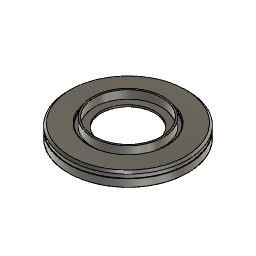
TouchCap (Autodesk Fusion 360 design; units mm, degrees)
Autodesk Fusion 360 part; units mm, degrees
sketch "Sketch2" plane through (0, 0, 0) normal (0, 1, 0) x (1, 0, 0) in component "LensCap_Sony20mm"
  line L0 (18.85, -1.2) -> (22.35, -1.2)
  line L1 (22.35, -1.2) -> (22.35, 0)
  line L2 (22.35, 0) -> (26, 0)
  line L3 (26, 0) -> (26, -2.7)
  line L4 (26, -2.7) -> (18.85, -2.7)
  line L5 (18.85, -2.7) -> (18.85, -1.2)
  line L6 (17.35, -5.2) -> (17.35, -1.2)
  line L7 (17.35, -1.2) -> (20.85, -1.2)
  line L8 (20.85, -1.2) -> (20.85, -0.2)
  line L9 (20.85, -0.2) -> (13.25, -0.2)
  line L10 (13.25, -0.2) -> (13.25, -1.2)
  line L11 (13.25, -1.2) -> (16.55, -1.2)
  line L12 (16.55, -1.2) -> (16.55, -5.2)
  line L13 (16.55, -5.2) -> (17.35, -5.2)
  line L14 (0, 0) -> (0, -2.7)
  line L15 (22.35, 0) -> (0, 0)
  line L16 (0, -2.7) -> (18.85, -2.7)
  line L17 (18.85, 0) -> (18.85, 2)
  line L18 (18.85, 2) -> (22.45, 2)
  line L19 (22.45, 2) -> (22.45, 5)
  line L20 (22.45, 5) -> (23.65, 5)
  line L21 (23.65, 5) -> (23.65, 2)
  line L22 (23.65, 2) -> (26, 2)
  line L23 (26, 2) -> (26, 0)
  dimension "d17" = 2.7
  dimension "d18" = 1.2
  dimension "d19" = 0.8
  dimension "d20" = 1
  dimension "d21" = 16.55
  dimension "d22" = 1.5
  dimension "d24" = 3.5
  dimension "d25" = 3.3
  dimension "d26" = 4
  dimension "d33" = 1.5
  dimension "d34" = 2
  dimension "d35" = 3
  dimension "d36" = 23.65
  dimension "d37" = 1.2
  dimension "d40" = 26
  constraint horizontal L0
  constraint perpendicular L0 L1
  constraint perpendicular L1 L2
  constraint perpendicular L2 L3
  constraint perpendicular L1 L4
  constraint perpendicular L4 L5
  constraint perpendicular L0 L6
  constraint perpendicular L6 L7
  constraint perpendicular L0 L8
  constraint perpendicular L8 L9
  constraint perpendicular L9 L10
  constraint perpendicular L10 L11
  constraint perpendicular L11 L12
  constraint perpendicular L6 L13
  constraint coincident L14.start L2
  constraint coincident L6.end L11
  constraint coincident L0 L7.end
  constraint coincident L14.start L15.end
  constraint horizontal L16
  constraint vertical L14
  constraint coincident L15 L17.start
  constraint perpendicular L15 L17
  constraint perpendicular L17 L18
  constraint perpendicular L18 L19
  constraint perpendicular L19 L20
  constraint perpendicular L20 L21
  constraint perpendicular L21 L22
  constraint perpendicular L22 L23
  constraint coincident L18 L21.end
  constraint coincident L0.start L17
  measures "d17" distance of L3.end L2.end
  measures "d18" distance of L0.end L1.end
  measures "d19" distance of L6.start L12.end
  measures "d20" distance of L7.end L8.end
  measures "d21" horizontal distance of L14.start L12.end
  measures "d22" horizontal distance of L4.end L6.start
  measures "d24" horizontal distance of L6.end L8.end
  measures "d25" horizontal distance of L9.end L11.end
  measures "d26" distance of L11.end L12.end
  measures "d33" distance of L1 L8
  measures "d34" distance of L22.end L2.end
  measures "d35" distance of L20.end L21.end
  measures "d36" distance of L14.start L21
  measures "d37" distance of L19.end L20.end
  measures "d40" distance of L14.start L2.end
revolve "Revolve3" add sketch "Sketch2" angle 360 about axis through (0, 0, 1.75) along (0, 0, 1) contours L0 L1 L2 L3 L4 L5 L7 makes body 1 in component "LensCap_Sony20mm"
revolve "Revolve4" add sketch "Sketch2" angle 360 about axis through (0, 0, 1.75) along (0, 0, 1) separate body contours L2 L15 L17 L18 L19 L20 L21 L22 L23 makes body 2 in component "LensCap_Sony20mm"
revolve "Revolve5" add sketch "Sketch2" angle 360 about axis through (0, 0, 1.75) along (0, 0, 1) separate body contours L0 L6 L7 L8 L9 L10 L11 L12 L16 | L6 L12 L13 L16 makes body 3 in component "LensCap_Sony20mm"
chamfer "Chamfer5" distance 1 angle 45 1 edges at (-24.2405, -9.402, 2.7) on bodies 1 in component "LensCap_Sony20mm"
sketch "Sketch3" plane through (0, 0, 0) normal (0, 0, 1) x (1, 0, 0) in component "LensCap_Sony20mm"
  circle A0 centre (0, 0) radius 26 construction
  circle A1 centre (0, 0) radius 22.35 construction
  line L0 (22.35, 0) -> (26, 0) construction
  circle A2 centre (0, 0) radius 24.175 construction
  line L1 (0, 0) -> (0, 26) construction
  circle A3 centre (0, 24.175) radius 0.8
  circle A4 centre (-20.9362, -12.0875) radius 0.8
  circle A5 centre (20.9362, -12.0875) radius 0.8
  circle A6 centre (0, 24.175) radius 0.95
  circle A7 centre (-20.9362, -12.0875) radius 0.95
  circle A8 centre (20.9362, -12.0875) radius 0.95
  point P0 (26, 0)
  point P1 (22.35, 0)
  point P2 (24.175, 0)
  dimension "d46" = 360
  dimension "d47" = 1.6
  dimension "d48" = 0.15
  constraint coincident A0.centre A1.centre
  constraint concentric A0 A1
  constraint coincident A1 P1
  constraint coincident A0 P0
  constraint coincident P1 L0.start
  constraint coincident P0 L0.end
  constraint coincident A0 L1.end
  constraint vertical L1
  constraint midpoint L0 P2
  constraint coincident A2 P2
  constraint coincident A2 A3.centre
  constraint coincident L1 A3.centre
  measures "d47" diameter of A3
extrude "Extrude5" add sketch "Sketch3" against normal blind 1.8 contours A3 | A4 | A5 bodies 1 in component "LensCap_Sony20mm"
extrude "Extrude6" cut sketch "Sketch3" against normal up to surface (2 mm away) contours A3 | A4 | A5 | A6 | A7 | A8 bodies 2 in component "LensCap_Sony20mm"
chamfer "Chamfer9" distance 0.3 angle 45 3 edges at (0, 23.65, -2) (-20.4815, -11.825, -2) (20.4815, -11.825, -2) on bodies 2 in component "LensCap_Sony20mm"
chamfer "Chamfer10" distance 0.3 angle 45 1 edges at (-17.5744, -6.8165, 2.7) on bodies 1 in component "LensCap_Sony20mm"
chamfer "Chamfer7" distance 0.25 angle 45 1 faces at (18.239, -1.0358, 0.2) on bodies 3 in component "LensCap_Sony20mm"
chamfer "Chamfer8" distance 0.25 angle 45 1 faces at (-3.5989, 22.4717, 0) on bodies 2 in component "LensCap_Sony20mm"
sketch "Sketch1" plane through (0, 0, 0) normal (0, 1, 0) x (1, 0, 0) in component "Blob"
  line L0 (0, 0) -> (0, -24.5001)
  line L1 (-13.5, 0) -> (-13.5, -3)
  ellipse E0 centre (17.5, -12.055) end of major axis (17.5, -18.055) minor radius 2.5
  line L2 (17.5, -6.055) -> (17.5, -18.055)
  line L3 (15, -12.055) -> (20, -12.055)
  circle A0 centre (0, 5.4999) radius 30
  line L4 (-13.5, -3) -> (-10, -3)
  line L5 (-10, -3) -> (-10, -5)
  line L6 (0, 5.4999) -> (0, 0) construction
  line L7 (-10, -5) -> (0, -5)
  line L8 (-16.5, 0) -> (-13.5, 0)
  line L9 (-16.5, 0) -> (-16.5, -19.555)
  ellipse E1 centre (-17.5, -12.055) end of major axis (-17.5, -6.055) minor radius 2.5
  line L10 (-17.5, -18.055) -> (-17.5, -6.055)
  line L11 (-15, -12.055) -> (-20, -12.055)
  circle A1 centre (0, -8.5) radius 7.5
  dimension "d683" = 3
  dimension "d684" = 3.5
  dimension "d685" = 15
  dimension "d686" = 16.5
  dimension "d687" = 3
  dimension "d688" = 2
  dimension "d689" = 8.5
  dimension "d690" = 19.555
  dimension "d691" = 60
  dimension "d697" = 1
  dimension "d698" = 7.5
  dimension "d699" = 12
  dimension "d700" = 5
  constraint horizontal L8
  constraint perpendicular L1 L8
  constraint perpendicular L1 L4
  constraint perpendicular L4 L5
  constraint perpendicular L5 L7
  constraint coincident L9.end A0
  constraint perpendicular L8 L9
  constraint coincident L0.start L6.end
  constraint coincident L0.end A0
  constraint perpendicular L0 L8
  constraint coincident L7.end L0
  constraint coincident A0.centre L6.start
  constraint coincident L0.start L8
  constraint vertical L6
  constraint coincident A1.centre L0
  constraint coincident L10.start E1
  constraint coincident L10.end E1
  constraint coincident L11.start E1
  constraint coincident L11.end E1
  constraint parallel L9 L10
  constraint coincident L2.start E0
  constraint coincident L2.end E0
  constraint coincident L3.start E0
  constraint coincident L3.end E0
  constraint vertical L2
  constraint symmetric L0 L2 L10
  constraint symmetric L0 L3 L11
  constraint symmetric L10.start L2.end L0
  constraint symmetric L11.start L3.start L0
  measures "d683" distance of L8.start L1.start
  measures "d684" distance of L1.end L4.end
  measures "d685" diameter of A1
  measures "d686" distance of L8.start L0.start
  measures "d687" distance of L1.start L1.end
  measures "d688" distance of L4.end L5.end
  measures "d689" distance of A1.centre L0.start
  measures "d690" distance of L8.start L9.end
  measures "d691" diameter of A0
  measures "d697" horizontal distance of L9.end L10.start
  measures "d698" distance of L9.end E1.centre
  measures "d699" distance of E1
revolve "Revolve1" add sketch "Sketch1" angle 360 about axis through (0, 0, 0) along (0, 0, 1) separate body contours L0 L7 A1 | L0 L7 A1 | L0 L1 A0 L4 L5 L7 L8 L9 E1 A1 | L9 E1 L11 | L9 E1 L11 picked at (-11.3366, -16.9039) makes body 4 in component "Blob"
extrude "Extrude1" cut sketch "Sketch1" along normal through all and the other way through all contours L9 E1 L10 L11 | L9 E1 L11 | L9 E1 L10 L11 | L9 E1 L11 | E1 L10 L11 | E1 L10 L11 | E0 L2 L3 | E0 L2 L3 | E0 L2 L3 | E0 L2 L3 bodies 4 in component "Blob"
sketch "Sketch2 (2)" plane through (0, 0, 0) normal (0, 1, 0) x (1, 0, 0) in component "LensCap_Sony20mm_2"
  line L0 (18.6, -1.2) -> (24.4, -1.2)
  line L1 (24.4, -1.2) -> (24.4, 0)
  line L2 (24.4, 0) -> (29, 0)
  line L3 (29, 0) -> (29, -2.7)
  line L4 (29, -2.7) -> (18.6, -2.7)
  line L5 (18.6, -2.7) -> (18.6, -1.2)
  line L6 (17.1, -5.2) -> (17.1, -1.2)
  line L7 (17.1, -1.2) -> (20.4, -1.2)
  line L8 (20.4, -1.2) -> (20.4, -0.2)
  line L9 (20.4, -0.2) -> (13, -0.2)
  line L10 (13, -0.2) -> (13, -1.2)
  line L11 (13, -1.2) -> (16.3, -1.2)
  line L12 (16.3, -1.2) -> (16.3, -5.2)
  line L13 (16.3, -5.2) -> (17.1, -5.2)
  line L14 (0, 0) -> (0, -2.7)
  line L15 (24.4, 0) -> (0, 0)
  line L16 (0, -2.7) -> (18.6, -2.7)
  line L17 (18.6, 0) -> (18.6, 1)
  line L18 (18.6, 1) -> (26.65, 1)
  line L19 (26.65, 1) -> (26.65, 4)
  line L20 (26.65, 4) -> (28.25, 4)
  line L21 (28.25, 4) -> (28.25, 1)
  line L22 (28.25, 1) -> (29, 1)
  line L23 (29, 1) -> (29, 0)
  line L24 (28.25, 4) -> (29, 4)
  line L25 (29, 4) -> (29, 1)
  dimension "d17_1" = 2.7
  dimension "d18_1" = 1.2
  dimension "d19_1" = 0.8
  dimension "d20_1" = 1
  dimension "d21_1" = 16.3
  dimension "d22_1" = 1.5
  dimension "d24_1" = 3.3
  dimension "d25_1" = 3.3
  dimension "d26_1" = 4
  dimension "d33_1" = 4
  dimension "d34_1" = 1
  dimension "d35_1" = 3
  dimension "d37_1" = 1.6
  dimension "d40_1" = 29
  dimension "d77" = 26.65
  dimension "d78" = 28.25
  constraint horizontal L0
  constraint perpendicular L0 L1
  constraint perpendicular L1 L2
  constraint perpendicular L2 L3
  constraint perpendicular L1 L4
  constraint perpendicular L4 L5
  constraint perpendicular L0 L6
  constraint perpendicular L6 L7
  constraint perpendicular L0 L8
  constraint perpendicular L8 L9
  constraint perpendicular L9 L10
  constraint perpendicular L10 L11
  constraint perpendicular L11 L12
  constraint perpendicular L6 L13
  constraint coincident L14.start L2
  constraint coincident L6.end L11
  constraint coincident L0 L7.end
  constraint coincident L14.start L15.end
  constraint horizontal L16
  constraint vertical L14
  constraint coincident L15 L17.start
  constraint perpendicular L15 L17
  constraint perpendicular L17 L18
  constraint perpendicular L18 L19
  constraint perpendicular L19 L20
  constraint perpendicular L20 L21
  constraint perpendicular L21 L22
  constraint perpendicular L22 L23
  constraint coincident L18 L21.end
  constraint coincident L0.start L17
  constraint perpendicular L21 L24
  constraint perpendicular L24 L25
  measures "d17_1" distance of L3.end L2.end
  measures "d18_1" distance of L0.end L1.end
  measures "d19_1" distance of L6.start L12.end
  measures "d20_1" distance of L7.end L8.end
  measures "d21_1" horizontal distance of L14.start L12.end
  measures "d22_1" horizontal distance of L4.end L6.start
  measures "d24_1" horizontal distance of L6.end L8.end
  measures "d25_1" horizontal distance of L9.end L11.end
  measures "d26_1" distance of L11.end L12.end
  measures "d33_1" distance of L1 L8
  measures "d34_1" distance of L22.end L2.end
  measures "d35_1" distance of L20.end L21.end
  measures "d37_1" distance of L19.end L20.end
  measures "d40_1" distance of L14.start L2.end
  measures "d77" horizontal distance of L14.start L19.end
  measures "d78" horizontal distance of L14.start L20.end
revolve "Revolve3'" add sketch "Sketch2 (2)" angle 360 about axis through (0, 0, 1.75) along (0, 0, 1) separate body contours L0 L1 L2 L3 L4 L5 L7 makes body 5 in component "LensCap_Sony20mm_2"
revolve "Revolve4'" add sketch "Sketch2 (2)" angle 360 about axis through (0, 0, 1.75) along (0, 0, 1) separate body contours L2 L15 L17 L18 L19 L20 L21 L22 L23 | L21 L22 L24 L25 makes body 6 in component "LensCap_Sony20mm_2"
revolve "Revolve5'" add sketch "Sketch2 (2)" angle 360 about axis through (0, 0, 1.75) along (0, 0, 1) separate body contours L0 L6 L7 L8 L9 L10 L11 L12 L16 | L6 L12 L13 L16 makes body 7 in component "LensCap_Sony20mm_2"
chamfer "Chamfer5'" distance 1 angle 45 1 edges at (-27.0375, -10.4868, 2.7) on bodies 5 in component "LensCap_Sony20mm_2"
sketch "Sketch3 (2)" plane through (0, 0, 0) normal (0, 0, 1) x (1, 0, 0) in component "LensCap_Sony20mm_2"
  circle A0 centre (0, 0) radius 29 construction
  circle A1 centre (0, 0) radius 24.4 construction
  line L0 (24.4, 0) -> (29, 0) construction
  circle A2 centre (0, 0) radius 26.7 construction
  line L1 (0, 0) -> (0, 29) construction
  circle A3 centre (0, 0) radius 20.4
  circle A4 centre (0, 0) radius 24.8 construction
  line L2 (0, 0) -> (24.8, 0) construction
  line L3 (0, 0) -> (22.4764, -10.4809) construction
  circle A5 centre (14.2796, -6.6587) radius 9.0442 construction
  circle A6 centre (14.2796, -6.6587) radius 7.8442 construction
  circle A7 centre (21.9326, -10.2274) radius 0.6
  arc A8 (22.4764, -10.4809) -> (20.4, 0) centre (14.2796, -6.6587) ccw
  arc A9 (21.3889, -9.9738) -> (20.3317, -1.6683) centre (14.2796, -6.6587) ccw
  arc A10 (23.5102, 2.0569) -> (18.4419, 8.721) centre (15.6959, 1.3732) ccw
  arc A11 (24.7056, 2.1615) -> (17.6669, 10.2) centre (15.6959, 1.3732) ccw
  circle A12 centre (24.1079, 2.1092) radius 0.6
  arc A13 (19.332, 13.5364) -> (11.6106, 16.7736) centre (12.9064, 9.0372) ccw
  arc A14 (20.315, 14.2247) -> (10.2, 17.6669) centre (12.9064, 9.0372) ccw
  circle A15 centre (19.8235, 13.8805) radius 0.6
  arc A16 (9.9738, 21.3889) -> (1.6683, 20.3317) centre (6.6587, 14.2796) ccw
  arc A17 (10.4809, 22.4764) -> (0, 20.4) centre (6.6587, 14.2796) ccw
  circle A18 centre (10.2274, 21.9326) radius 0.6
  arc A19 (-2.0569, 23.5102) -> (-8.721, 18.4419) centre (-1.3732, 15.6959) ccw
  arc A20 (-2.1615, 24.7056) -> (-10.2, 17.6669) centre (-1.3732, 15.6959) ccw
  circle A21 centre (-2.1092, 24.1079) radius 0.6
  arc A22 (-13.5364, 19.332) -> (-16.7736, 11.6106) centre (-9.0372, 12.9064) ccw
  arc A23 (-14.2247, 20.315) -> (-17.6669, 10.2) centre (-9.0372, 12.9064) ccw
  circle A24 centre (-13.8805, 19.8235) radius 0.6
  circle A25 centre (14.2796, -6.6587) radius 7.4442 construction
  circle A26 centre (20.1774, -1.7955) radius 0.2
  circle A27 centre (18.3719, 8.5337) radius 0.2
  circle A28 centre (11.6437, 16.5763) radius 0.2
  circle A29 centre (1.7955, 20.1774) radius 0.2
  circle A30 centre (-8.5337, 18.3719) radius 0.2
  circle A31 centre (-16.5763, 11.6437) radius 0.2
  arc A32 (20.2758, -2.2472) -> (20.0231, -1.9228) centre (14.2796, -6.6587) ccw
  arc A33 (18.683, 8.1918) -> (18.3019, 8.3463) centre (15.6959, 1.3732) ccw
  arc A34 (12.0841, 16.4358) -> (11.6767, 16.3791) centre (12.9064, 9.0372) ccw
  arc A35 (2.2472, 20.2758) -> (1.9228, 20.0231) centre (6.6587, 14.2796) ccw
  arc A36 (-8.1918, 18.683) -> (-8.3463, 18.3019) centre (-1.3732, 15.6959) ccw
  arc A37 (-16.4358, 12.0841) -> (-16.3791, 11.6767) centre (-9.0372, 12.9064) ccw
  arc A38 (-21.3889, 9.9738) -> (-20.3317, 1.6683) centre (-14.2796, 6.6587) ccw
  arc A39 (-22.4764, 10.4809) -> (-20.4, 0) centre (-14.2796, 6.6587) ccw
  circle A40 centre (-21.9326, 10.2274) radius 0.6
  arc A41 (-20.2758, 2.2472) -> (-20.0231, 1.9228) centre (-14.2796, 6.6587) ccw
  circle A42 centre (-20.1774, 1.7955) radius 0.2
  arc A43 (-23.5102, -2.0569) -> (-18.4419, -8.721) centre (-15.6959, -1.3732) ccw
  arc A44 (-24.7056, -2.1615) -> (-17.6669, -10.2) centre (-15.6959, -1.3732) ccw
  circle A45 centre (-24.1079, -2.1092) radius 0.6
  arc A46 (-18.683, -8.1918) -> (-18.3019, -8.3463) centre (-15.6959, -1.3732) ccw
  circle A47 centre (-18.3719, -8.5337) radius 0.2
  arc A48 (-19.332, -13.5364) -> (-11.6106, -16.7736) centre (-12.9064, -9.0372) ccw
  arc A49 (-20.315, -14.2247) -> (-10.2, -17.6669) centre (-12.9064, -9.0372) ccw
  circle A50 centre (-19.8235, -13.8805) radius 0.6
  arc A51 (-12.0841, -16.4358) -> (-11.6767, -16.3791) centre (-12.9064, -9.0372) ccw
  circle A52 centre (-11.6437, -16.5763) radius 0.2
  arc A53 (-9.9738, -21.3889) -> (-1.6683, -20.3317) centre (-6.6587, -14.2796) ccw
  arc A54 (-10.4809, -22.4764) -> (0, -20.4) centre (-6.6587, -14.2796) ccw
  circle A55 centre (-10.2274, -21.9326) radius 0.6
  arc A56 (-2.2472, -20.2758) -> (-1.9228, -20.0231) centre (-6.6587, -14.2796) ccw
  circle A57 centre (-1.7955, -20.1774) radius 0.2
  arc A58 (2.0569, -23.5102) -> (8.721, -18.4419) centre (1.3732, -15.6959) ccw
  arc A59 (2.1615, -24.7056) -> (10.2, -17.6669) centre (1.3732, -15.6959) ccw
  circle A60 centre (2.1092, -24.1079) radius 0.6
  arc A61 (8.1918, -18.683) -> (8.3463, -18.3019) centre (1.3732, -15.6959) ccw
  circle A62 centre (8.5337, -18.3719) radius 0.2
  arc A63 (13.5364, -19.332) -> (16.7736, -11.6106) centre (9.0372, -12.9064) ccw
  arc A64 (14.2247, -20.315) -> (17.6669, -10.2) centre (9.0372, -12.9064) ccw
  circle A65 centre (13.8805, -19.8235) radius 0.6
  arc A66 (16.4358, -12.0841) -> (16.3791, -11.6767) centre (9.0372, -12.9064) ccw
  circle A67 centre (16.5763, -11.6437) radius 0.2
  arc A68 (1.4635, 26.0089) -> (-1.4635, 26.0089) centre (0, 0) ccw
  arc A69 (1.4635, 26.0089) -> (1.5365, 27.3068) centre (1.5, 26.6578) ccw
  arc A70 (1.5365, 27.3068) -> (-1.5365, 27.3068) centre (0, 0) ccw
  arc A71 (-1.5365, 27.3068) -> (-1.4635, 26.0089) centre (-1.5, 26.6578) ccw
  arc A72 (1.5, 26.6578) -> (-1.5, 26.6578) centre (0, 0) ccw construction
  arc A73 (-1.5421, 27.4066) -> (-1.4579, 25.909) centre (-1.5, 26.6578) ccw
  arc A74 (1.4579, 25.909) -> (-1.4579, 25.909) centre (0, 0) ccw
  arc A75 (1.4579, 25.909) -> (1.5421, 27.4066) centre (1.5, 26.6578) ccw
  arc A76 (1.5421, 27.4066) -> (-1.5421, 27.4066) centre (0, 0) ccw
  arc A77 (-21.7089, 14.2171) -> (-23.1668, 11.692) centre (0, 0) ccw
  arc A78 (-21.7926, 14.2718) -> (-23.2561, 11.737) centre (0, 0) ccw
  arc A79 (-24.5059, 12.3678) -> (-23.1668, 11.692) centre (-23.8364, 12.0299) ccw
  arc A80 (-24.4166, 12.3227) -> (-23.2561, 11.737) centre (-23.8364, 12.0299) ccw
  arc A81 (-22.8801, 14.9841) -> (-24.4166, 12.3227) centre (0, 0) ccw
  arc A82 (-22.9638, 15.0389) -> (-24.5059, 12.3678) centre (0, 0) ccw
  arc A83 (-21.7926, 14.2718) -> (-22.8801, 14.9841) centre (-22.3364, 14.628) ccw
  arc A84 (-21.7089, 14.2171) -> (-22.9638, 15.0389) centre (-22.3364, 14.628) ccw
  arc A85 (-23.1668, -11.692) -> (-21.7089, -14.2171) centre (0, 0) ccw
  arc A86 (-23.2561, -11.737) -> (-21.7926, -14.2718) centre (0, 0) ccw
  arc A87 (-22.9638, -15.0389) -> (-21.7089, -14.2171) centre (-22.3364, -14.628) ccw
  arc A88 (-22.8801, -14.9841) -> (-21.7926, -14.2718) centre (-22.3364, -14.628) ccw
  arc A89 (-24.4166, -12.3227) -> (-22.8801, -14.9841) centre (0, 0) ccw
  arc A90 (-24.5059, -12.3678) -> (-22.9638, -15.0389) centre (0, 0) ccw
  arc A91 (-23.2561, -11.737) -> (-24.4166, -12.3227) centre (-23.8364, -12.0299) ccw
  arc A92 (-23.1668, -11.692) -> (-24.5059, -12.3678) centre (-23.8364, -12.0299) ccw
  arc A93 (-1.4579, -25.909) -> (1.4579, -25.909) centre (0, 0) ccw
  arc A94 (-1.4635, -26.0089) -> (1.4635, -26.0089) centre (0, 0) ccw
  arc A95 (1.5421, -27.4066) -> (1.4579, -25.909) centre (1.5, -26.6578) ccw
  arc A96 (1.5365, -27.3068) -> (1.4635, -26.0089) centre (1.5, -26.6578) ccw
  arc A97 (-1.5365, -27.3068) -> (1.5365, -27.3068) centre (0, 0) ccw
  arc A98 (-1.5421, -27.4066) -> (1.5421, -27.4066) centre (0, 0) ccw
  arc A99 (-1.4635, -26.0089) -> (-1.5365, -27.3068) centre (-1.5, -26.6578) ccw
  arc A100 (-1.4579, -25.909) -> (-1.5421, -27.4066) centre (-1.5, -26.6578) ccw
  arc A101 (21.7089, -14.2171) -> (23.1668, -11.692) centre (0, 0) ccw
  arc A102 (21.7926, -14.2718) -> (23.2561, -11.737) centre (0, 0) ccw
  arc A103 (24.5059, -12.3678) -> (23.1668, -11.692) centre (23.8364, -12.0299) ccw
  arc A104 (24.4166, -12.3227) -> (23.2561, -11.737) centre (23.8364, -12.0299) ccw
  arc A105 (22.8801, -14.9841) -> (24.4166, -12.3227) centre (0, 0) ccw
  arc A106 (22.9638, -15.0389) -> (24.5059, -12.3678) centre (0, 0) ccw
  arc A107 (21.7926, -14.2718) -> (22.8801, -14.9841) centre (22.3364, -14.628) ccw
  arc A108 (21.7089, -14.2171) -> (22.9638, -15.0389) centre (22.3364, -14.628) ccw
  arc A109 (23.1668, 11.692) -> (21.7089, 14.2171) centre (0, 0) ccw
  arc A110 (23.2561, 11.737) -> (21.7926, 14.2718) centre (0, 0) ccw
  arc A111 (22.9638, 15.0389) -> (21.7089, 14.2171) centre (22.3364, 14.628) ccw
  arc A112 (22.8801, 14.9841) -> (21.7926, 14.2718) centre (22.3364, 14.628) ccw
  arc A113 (24.4166, 12.3227) -> (22.8801, 14.9841) centre (0, 0) ccw
  arc A114 (24.5059, 12.3678) -> (22.9638, 15.0389) centre (0, 0) ccw
  arc A115 (23.2561, 11.737) -> (24.4166, 12.3227) centre (23.8364, 12.0299) ccw
  arc A116 (23.1668, 11.692) -> (24.5059, 12.3678) centre (23.8364, 12.0299) ccw
  point P0 (29, 0)
  point P1 (24.4, 0)
  point P2 (26.7, 0)
  point P3 (20.4, 0)
  point P4 (22.4764, -10.4809)
  point P5 (24.8, 0)
  point P6 (21.3889, -9.9738)
  dimension "d84" = 25
  dimension "d87" = -1.2
  dimension "d89" = 360
  dimension "d96" = -1.6
  dimension "d101" = 3
  dimension "d102" = 1.3
  dimension "d103" = -0.1
  dimension "d105" = 360
  dimension "d107" = 0.4
  constraint coincident A0.centre A1.centre
  constraint concentric A0 A1
  constraint coincident A1 P1
  constraint coincident A0 P0
  constraint coincident P1 L0.start
  constraint coincident P0 L0.end
  constraint coincident A0 L1.end
  constraint vertical L1
  constraint midpoint L0 P2
  constraint coincident A2 P2
  constraint coincident P3 A3
  constraint coincident A4 P5
  constraint horizontal L2
  constraint coincident A4 P4
  constraint coincident P4 L3.end
  constraint coincident P5 L2.end
  constraint coincident P3 A5
  constraint coincident P4 A5
  constraint coincident L3 A5.centre
  constraint coincident L3 A7.centre
  constraint tangent A4 A7
  constraint tangent A6 A7
  constraint coincident P3 A8.end
  constraint coincident A5.centre A6.centre
  constraint coincident A3 A9.end
  constraint coincident A6 A9.end
  constraint coincident A6 P6
  constraint coincident A7 P6
  constraint coincident P6 A9.start
  constraint tangent A25 A26
  constraint tangent A6 A26
  constraint coincident A9.end A26
  constraint coincident A26 A32.end
  constraint coincident A25 A32.end
  constraint coincident A3 A32.start
  constraint tangent A68 A69
  constraint tangent A69 A70
  constraint tangent A70 A71
  constraint tangent A68 A71
  constraint coincident A2 A69.centre
  constraint symmetric L1 A71.centre A69.centre
  measures "d84" angle of L2 L3
  measures "d101" distance of A71.centre A69.centre
  measures "d102" distance of A68.start A69.end
extrude "Extrude5'" add sketch "Sketch3 (2)" against normal up to surface (0.8 mm away) contours A68 A69 A70 A71 | A78 A80 A81 A83 | A86 A88 A89 A91 | A94 A96 A97 A99 | A102 A104 A105 A107 | A110 A112 A113 A115 bodies 5 in component "LensCap_Sony20mm_2"
extrude "Extrude6'" cut sketch "Sketch3 (2)" against normal up to surface (1 mm away) contours A68 A69 A70 A71 | A73 A74 A75 A76 | A77 A79 A82 A84 | A78 A80 A81 A83 | A85 A87 A90 A92 | A86 A88 A89 A91 | A93 A95 A98 A100 | A94 A96 A97 A99 | A101 A103 A106 A108 | A102 A104 A105 A107 | A109 A111 A114 A116 | A110 A112 A113 A115 bodies 6 in component "LensCap_Sony20mm_2"
extrude "Extrude7" add sketch "Sketch3 (2)" along normal up to surface (1 mm away) from surface at 0.2 contours A3 A7 A8 A9 | A7 | A3 A10 A11 A12 | A12 | A3 A63 A64 A65 | A65 | A3 A13 A14 A15 | A15 | A3 A58 A59 A60 | A60 | A3 A16 A17 A18 | A18 | A3 A53 A54 A55 | A55 | A3 A19 A20 A21 | A21 | A3 A48 A49 A50 | A50 | A3 A22 A23 A24 | A24 | A3 A43 A44 A45 | A45 | A3 A38 A39 A40 | A40 bodies 7 in component "LensCap_Sony20mm_2"
extrude "Extrude8" cut sketch "Sketch3 (2)" along normal up to surface (1 mm away) from surface at 0.2 contours A3 A27 A33 | A3 A26 | A3 A27 | A3 A26 A32 | A3 A28 A34 | A3 A67 | A3 A67 | A3 A28 | A3 A66 A67 | A3 A29 A35 | A3 A62 | A3 A29 | A3 A61 A62 | A3 A30 A36 | A3 A57 | A3 A30 | A3 A56 A57 | A3 A31 A37 | A3 A52 | A3 A31 | A3 A51 A52 | A3 A41 A42 | A3 A47 | A3 A42 | A3 A46 A47 picked at (20.2057, -1.8001) picked at (18.3987, 8.5439) picked at (11.6618, 16.5986) picked at (8.543, -18.3991) picked at (1.8001, 20.2057) picked at (-1.7935, -20.2064) picked at (-8.5439, 18.3987) picked at (-11.6631, -16.5977) picked at (-16.5991, 11.661) picked at (-18.397, -8.5476) picked at (-20.2062, 1.7944) bodies 7 in component "LensCap_Sony20mm_2"
chamfer "Chamfer10'" distance 0.3 angle 45 1 edges at (-17.3413, -6.726, 2.7) on bodies 5 in component "LensCap_Sony20mm_2"
chamfer "Chamfer7'" distance 0.15 angle 45 1 faces at (13.516, -11.541, 0.2) on bodies 7 in component "LensCap_Sony20mm_2"
chamfer "Chamfer8'" distance 0.25 angle 45 1 faces at (25.4254, -1.4407, 0) on bodies 6 in component "LensCap_Sony20mm_2"
chamfer "Chamfer11" distance 0.25 angle 45 1 edges at (-17.3413, -6.726, -1) on bodies 6 in component "LensCap_Sony20mm_2"
chamfer "Chamfer12" distance 0.2 angle 45 1 faces at (28.1087, -1.4407, -4) on bodies 6 in component "LensCap_Sony20mm_2"
chamfer "Chamfer13" distance 0.2 angle 45 1 edges at (-17.3413, -6.726, 1.2) on bodies 5 in component "LensCap_Sony20mm_2"
chamfer "Chamfer14" distance 0.4 angle 45 6 edges at (-23.0796, 13.325, -1) (-23.0796, -13.325, -1) (0, 26.65, -1) (0, -26.65, -1) (23.0796, -13.325, -1) (23.0796, 13.325, -1) on bodies 6 in component "LensCap_Sony20mm_2"
chamfer "Chamfer15" distance 0.4 angle 45 1 edges at (-22.7488, -8.8234, 0) on bodies 5 in component "LensCap_Sony20mm_2"
sketch "Sketch2 (3)" plane through (0, 0, 0) normal (0, 1, 0) x (1, 0, 0) in component "LensCap_Pergear10mm"
  line L0 (18.6, -1.2) -> (24.4, -1.2)
  line L1 (24.4, -1.2) -> (24.4, 0)
  line L2 (24.4, 0) -> (31, 0)
  line L3 (31, 0) -> (31, -2.7)
  line L4 (31, -2.7) -> (18.6, -2.7)
  line L5 (18.6, -2.7) -> (18.6, -1.2)
  line L6 (17.1, -5.2) -> (17.1, -1.2)
  line L7 (17.1, -1.2) -> (20.4, -1.2)
  line L8 (20.4, -1.2) -> (20.4, -0.2)
  line L9 (20.4, -0.2) -> (13, -0.2)
  line L10 (13, -0.2) -> (13, -1.2)
  line L11 (13, -1.2) -> (16.3, -1.2)
  line L12 (16.3, -1.2) -> (16.3, -5.2)
  line L13 (16.3, -5.2) -> (17.1, -5.2)
  line L14 (0, 0) -> (0, -2.7)
  line L15 (24.4, 0) -> (0, 0)
  line L16 (0, -2.7) -> (18.6, -2.7)
  line L17 (18.6, 0) -> (18.6, 1)
  line L18 (18.6, 1) -> (29, 1)
  line L19 (29, 1) -> (29, 7)
  line L20 (29, 7) -> (31, 7)
  line L21 (31, 7) -> (31, 0)
  dimension "d17_1_1" = 2.7
  dimension "d18_1_1" = 1.2
  dimension "d19_1_1" = 0.8
  dimension "d20_1_1" = 1
  dimension "d21_1_1" = 16.3
  dimension "d22_1_1" = 1.5
  dimension "d24_1_1" = 3.3
  dimension "d25_1_1" = 3.3
  dimension "d26_1_1" = 4
  dimension "d33_1_1" = 4
  dimension "d77_1" = 29
  dimension "d78_1" = 31
  dimension "d111" = 1
  dimension "d112" = 6
  dimension "d113" = 2
  constraint horizontal L0
  constraint perpendicular L0 L1
  constraint perpendicular L1 L2
  constraint perpendicular L2 L3
  constraint perpendicular L1 L4
  constraint perpendicular L4 L5
  constraint perpendicular L0 L6
  constraint perpendicular L6 L7
  constraint perpendicular L0 L8
  constraint perpendicular L8 L9
  constraint perpendicular L9 L10
  constraint perpendicular L10 L11
  constraint perpendicular L11 L12
  constraint perpendicular L6 L13
  constraint coincident L14.start L2
  constraint coincident L6.end L11
  constraint coincident L0 L7.end
  constraint coincident L14.start L15.end
  constraint horizontal L16
  constraint vertical L14
  constraint coincident L15 L17.start
  constraint perpendicular L15 L17
  constraint perpendicular L17 L18
  constraint perpendicular L18 L19
  constraint perpendicular L19 L20
  constraint coincident L0.start L17
  constraint perpendicular L20 L21
  constraint coincident L2.end L3.start
  measures "d17_1_1" distance of L3.end L2.end
  measures "d18_1_1" distance of L0.end L1.end
  measures "d19_1_1" distance of L6.start L12.end
  measures "d20_1_1" distance of L7.end L8.end
  measures "d21_1_1" horizontal distance of L14.start L12.end
  measures "d22_1_1" horizontal distance of L4.end L6.start
  measures "d24_1_1" horizontal distance of L6.end L8.end
  measures "d25_1_1" horizontal distance of L9.end L11.end
  measures "d26_1_1" distance of L11.end L12.end
  measures "d33_1_1" distance of L1 L8
  measures "d77_1" horizontal distance of L14.start L19.end
  measures "d78_1" horizontal distance of L14.start L20.end
  measures "d111" distance of L18 L2.end
  measures "d112" distance of L18.end L19.end
  measures "d113" distance of L19.end L20.end
revolve "Revolve3''" add sketch "Sketch2 (3)" angle 360 about axis through (0, 0, 1.75) along (0, 0, 1) separate body contours L0 L1 L2 L3 L4 L5 L7 makes body 8 in component "LensCap_Pergear10mm"
revolve "Revolve4''" add sketch "Sketch2 (3)" angle 360 about axis through (0, 0, 1.75) along (0, 0, 1) separate body contours L2 L15 L17 L18 L19 L20 L21 makes body 9 in component "LensCap_Pergear10mm"
revolve "Revolve5''" add sketch "Sketch2 (3)" angle 360 about axis through (0, 0, 1.75) along (0, 0, 1) separate body contours L0 L6 L7 L8 L9 L10 L11 L12 L16 | L6 L12 L13 L16 makes body 10 in component "LensCap_Pergear10mm"
chamfer "Chamfer5''" distance 1 angle 45 1 edges at (-28.9021, -11.2101, 2.7) on bodies 8 in component "LensCap_Pergear10mm"
sketch "Sketch3 (3)" plane through (0, 0, 0) normal (0, 0, 1) x (1, 0, 0) in component "LensCap_Pergear10mm"
  circle A0 centre (0, 0) radius 31 construction
  circle A1 centre (0, 0) radius 24.4 construction
  line L0 (24.4, 0) -> (31, 0) construction
  circle A2 centre (0, 0) radius 27.7 construction
  line L1 (0, 0) -> (0, 31) construction
  circle A3 centre (0, 0) radius 20.4
  circle A4 centre (0, 0) radius 24.8 construction
  line L2 (0, 0) -> (24.8, 0) construction
  line L3 (0, 0) -> (22.4764, -10.4809) construction
  circle A5 centre (14.2796, -6.6587) radius 9.0442 construction
  circle A6 centre (14.2796, -6.6587) radius 7.8442 construction
  circle A7 centre (21.9326, -10.2274) radius 0.6
  arc A8 (22.4764, -10.4809) -> (20.4, 0) centre (14.2796, -6.6587) ccw
  arc A9 (21.3889, -9.9738) -> (20.3317, -1.6683) centre (14.2796, -6.6587) ccw
  arc A10 (23.5102, 2.0569) -> (18.4419, 8.721) centre (15.6959, 1.3732) ccw
  arc A11 (24.7056, 2.1615) -> (17.6669, 10.2) centre (15.6959, 1.3732) ccw
  circle A12 centre (24.1079, 2.1092) radius 0.6
  arc A13 (19.332, 13.5364) -> (11.6106, 16.7736) centre (12.9064, 9.0372) ccw
  arc A14 (20.315, 14.2247) -> (10.2, 17.6669) centre (12.9064, 9.0372) ccw
  circle A15 centre (19.8235, 13.8805) radius 0.6
  arc A16 (9.9738, 21.3889) -> (1.6683, 20.3317) centre (6.6587, 14.2796) ccw
  arc A17 (10.4809, 22.4764) -> (0, 20.4) centre (6.6587, 14.2796) ccw
  circle A18 centre (10.2274, 21.9326) radius 0.6
  arc A19 (-2.0569, 23.5102) -> (-8.721, 18.4419) centre (-1.3732, 15.6959) ccw
  arc A20 (-2.1615, 24.7056) -> (-10.2, 17.6669) centre (-1.3732, 15.6959) ccw
  circle A21 centre (-2.1092, 24.1079) radius 0.6
  arc A22 (-13.5364, 19.332) -> (-16.7736, 11.6106) centre (-9.0372, 12.9064) ccw
  arc A23 (-14.2247, 20.315) -> (-17.6669, 10.2) centre (-9.0372, 12.9064) ccw
  circle A24 centre (-13.8805, 19.8235) radius 0.6
  circle A25 centre (14.2796, -6.6587) radius 7.4442 construction
  circle A26 centre (20.1774, -1.7955) radius 0.2
  circle A27 centre (18.3719, 8.5337) radius 0.2
  circle A28 centre (11.6437, 16.5763) radius 0.2
  circle A29 centre (1.7955, 20.1774) radius 0.2
  circle A30 centre (-8.5337, 18.3719) radius 0.2
  circle A31 centre (-16.5763, 11.6437) radius 0.2
  arc A32 (20.2758, -2.2472) -> (20.0231, -1.9228) centre (14.2796, -6.6587) ccw
  arc A33 (18.683, 8.1918) -> (18.3019, 8.3463) centre (15.6959, 1.3732) ccw
  arc A34 (12.0841, 16.4358) -> (11.6767, 16.3791) centre (12.9064, 9.0372) ccw
  arc A35 (2.2472, 20.2758) -> (1.9228, 20.0231) centre (6.6587, 14.2796) ccw
  arc A36 (-8.1918, 18.683) -> (-8.3463, 18.3019) centre (-1.3732, 15.6959) ccw
  arc A37 (-16.4358, 12.0841) -> (-16.3791, 11.6767) centre (-9.0372, 12.9064) ccw
  arc A38 (-21.3889, 9.9738) -> (-20.3317, 1.6683) centre (-14.2796, 6.6587) ccw
  arc A39 (-22.4764, 10.4809) -> (-20.4, 0) centre (-14.2796, 6.6587) ccw
  circle A40 centre (-21.9326, 10.2274) radius 0.6
  arc A41 (-20.2758, 2.2472) -> (-20.0231, 1.9228) centre (-14.2796, 6.6587) ccw
  circle A42 centre (-20.1774, 1.7955) radius 0.2
  arc A43 (-23.5102, -2.0569) -> (-18.4419, -8.721) centre (-15.6959, -1.3732) ccw
  arc A44 (-24.7056, -2.1615) -> (-17.6669, -10.2) centre (-15.6959, -1.3732) ccw
  circle A45 centre (-24.1079, -2.1092) radius 0.6
  arc A46 (-18.683, -8.1918) -> (-18.3019, -8.3463) centre (-15.6959, -1.3732) ccw
  circle A47 centre (-18.3719, -8.5337) radius 0.2
  arc A48 (-19.332, -13.5364) -> (-11.6106, -16.7736) centre (-12.9064, -9.0372) ccw
  arc A49 (-20.315, -14.2247) -> (-10.2, -17.6669) centre (-12.9064, -9.0372) ccw
  circle A50 centre (-19.8235, -13.8805) radius 0.6
  arc A51 (-12.0841, -16.4358) -> (-11.6767, -16.3791) centre (-12.9064, -9.0372) ccw
  circle A52 centre (-11.6437, -16.5763) radius 0.2
  arc A53 (-9.9738, -21.3889) -> (-1.6683, -20.3317) centre (-6.6587, -14.2796) ccw
  arc A54 (-10.4809, -22.4764) -> (0, -20.4) centre (-6.6587, -14.2796) ccw
  circle A55 centre (-10.2274, -21.9326) radius 0.6
  arc A56 (-2.2472, -20.2758) -> (-1.9228, -20.0231) centre (-6.6587, -14.2796) ccw
  circle A57 centre (-1.7955, -20.1774) radius 0.2
  arc A58 (2.0569, -23.5102) -> (8.721, -18.4419) centre (1.3732, -15.6959) ccw
  arc A59 (2.1615, -24.7056) -> (10.2, -17.6669) centre (1.3732, -15.6959) ccw
  circle A60 centre (2.1092, -24.1079) radius 0.6
  arc A61 (8.1918, -18.683) -> (8.3463, -18.3019) centre (1.3732, -15.6959) ccw
  circle A62 centre (8.5337, -18.3719) radius 0.2
  arc A63 (13.5364, -19.332) -> (16.7736, -11.6106) centre (9.0372, -12.9064) ccw
  arc A64 (14.2247, -20.315) -> (17.6669, -10.2) centre (9.0372, -12.9064) ccw
  circle A65 centre (13.8805, -19.8235) radius 0.6
  arc A66 (16.4358, -12.0841) -> (16.3791, -11.6767) centre (9.0372, -12.9064) ccw
  circle A67 centre (16.5763, -11.6437) radius 0.2
  arc A68 (1.4648, 27.0103) -> (-1.4648, 27.0103) centre (0, 0) ccw
  arc A69 (1.4648, 27.0103) -> (1.5352, 28.3084) centre (1.5, 27.6594) ccw
  arc A70 (1.5352, 28.3084) -> (-1.5352, 28.3084) centre (0, 0) ccw
  arc A71 (-1.5352, 28.3084) -> (-1.4648, 27.0103) centre (-1.5, 27.6594) ccw
  arc A72 (1.5, 27.6594) -> (-1.5, 27.6594) centre (0, 0) ccw construction
  arc A73 (-1.5406, 28.4083) -> (-1.4594, 26.9105) centre (-1.5, 27.6594) ccw
  arc A74 (1.4594, 26.9105) -> (-1.4594, 26.9105) centre (0, 0) ccw
  arc A75 (1.4594, 26.9105) -> (1.5406, 28.4083) centre (1.5, 27.6594) ccw
  arc A76 (1.5406, 28.4083) -> (-1.5406, 28.4083) centre (0, 0) ccw
  arc A77 (-22.5754, 14.7191) -> (-24.0348, 12.1914) centre (0, 0) ccw
  arc A78 (-22.6592, 14.7737) -> (-24.124, 12.2366) centre (0, 0) ccw
  arc A79 (-25.3726, 12.8699) -> (-24.0348, 12.1914) centre (-24.7037, 12.5306) ccw
  arc A80 (-25.2834, 12.8247) -> (-24.124, 12.2366) centre (-24.7037, 12.5306) ccw
  arc A81 (-23.7482, 15.4837) -> (-25.2834, 12.8247) centre (0, 0) ccw
  arc A82 (-23.832, 15.5383) -> (-25.3726, 12.8699) centre (0, 0) ccw
  arc A83 (-22.6592, 14.7737) -> (-23.7482, 15.4837) centre (-23.2037, 15.1287) ccw
  arc A84 (-22.5754, 14.7191) -> (-23.832, 15.5383) centre (-23.2037, 15.1287) ccw
  arc A85 (-24.0348, -12.1914) -> (-22.5754, -14.7191) centre (0, 0) ccw
  arc A86 (-24.124, -12.2366) -> (-22.6592, -14.7737) centre (0, 0) ccw
  arc A87 (-23.832, -15.5383) -> (-22.5754, -14.7191) centre (-23.2037, -15.1287) ccw
  arc A88 (-23.7482, -15.4837) -> (-22.6592, -14.7737) centre (-23.2037, -15.1287) ccw
  arc A89 (-25.2834, -12.8247) -> (-23.7482, -15.4837) centre (0, 0) ccw
  arc A90 (-25.3726, -12.8699) -> (-23.832, -15.5383) centre (0, 0) ccw
  arc A91 (-24.124, -12.2366) -> (-25.2834, -12.8247) centre (-24.7037, -12.5306) ccw
  arc A92 (-24.0348, -12.1914) -> (-25.3726, -12.8699) centre (-24.7037, -12.5306) ccw
  arc A93 (-1.4594, -26.9105) -> (1.4594, -26.9105) centre (0, 0) ccw
  arc A94 (-1.4648, -27.0103) -> (1.4648, -27.0103) centre (0, 0) ccw
  arc A95 (1.5406, -28.4083) -> (1.4594, -26.9105) centre (1.5, -27.6594) ccw
  arc A96 (1.5352, -28.3084) -> (1.4648, -27.0103) centre (1.5, -27.6594) ccw
  arc A97 (-1.5352, -28.3084) -> (1.5352, -28.3084) centre (0, 0) ccw
  arc A98 (-1.5406, -28.4083) -> (1.5406, -28.4083) centre (0, 0) ccw
  arc A99 (-1.4648, -27.0103) -> (-1.5352, -28.3084) centre (-1.5, -27.6594) ccw
  arc A100 (-1.4594, -26.9105) -> (-1.5406, -28.4083) centre (-1.5, -27.6594) ccw
  arc A101 (22.5754, -14.7191) -> (24.0348, -12.1914) centre (0, 0) ccw
  arc A102 (22.6592, -14.7737) -> (24.124, -12.2366) centre (0, 0) ccw
  arc A103 (25.3726, -12.8699) -> (24.0348, -12.1914) centre (24.7037, -12.5306) ccw
  arc A104 (25.2834, -12.8247) -> (24.124, -12.2366) centre (24.7037, -12.5306) ccw
  arc A105 (23.7482, -15.4837) -> (25.2834, -12.8247) centre (0, 0) ccw
  arc A106 (23.832, -15.5383) -> (25.3726, -12.8699) centre (0, 0) ccw
  arc A107 (22.6592, -14.7737) -> (23.7482, -15.4837) centre (23.2037, -15.1287) ccw
  arc A108 (22.5754, -14.7191) -> (23.832, -15.5383) centre (23.2037, -15.1287) ccw
  arc A109 (24.0348, 12.1914) -> (22.5754, 14.7191) centre (0, 0) ccw
  arc A110 (24.124, 12.2366) -> (22.6592, 14.7737) centre (0, 0) ccw
  arc A111 (23.832, 15.5383) -> (22.5754, 14.7191) centre (23.2037, 15.1287) ccw
  arc A112 (23.7482, 15.4837) -> (22.6592, 14.7737) centre (23.2037, 15.1287) ccw
  arc A113 (25.2834, 12.8247) -> (23.7482, 15.4837) centre (0, 0) ccw
  arc A114 (25.3726, 12.8699) -> (23.832, 15.5383) centre (0, 0) ccw
  arc A115 (24.124, 12.2366) -> (25.2834, 12.8247) centre (24.7037, 12.5306) ccw
  arc A116 (24.0348, 12.1914) -> (25.3726, 12.8699) centre (24.7037, 12.5306) ccw
  point P0 (31, 0)
  point P1 (24.4, 0)
  point P2 (27.7, 0)
  point P3 (20.4, 0)
  point P4 (22.4764, -10.4809)
  point P5 (24.8, 0)
  point P6 (21.3889, -9.9738)
  dimension "d84_1" = 25
  dimension "d87_1" = -1.2
  dimension "d89_1" = 360
  dimension "d96_1" = -1.6
  dimension "d101_1" = 3
  dimension "d102_1" = 1.3
  dimension "d103_1" = -0.1
  dimension "d105_1" = 360
  dimension "d107_1" = 0.4
  constraint coincident A0.centre A1.centre
  constraint concentric A0 A1
  constraint coincident A1 P1
  constraint coincident A0 P0
  constraint coincident P1 L0.start
  constraint coincident P0 L0.end
  constraint coincident A0 L1.end
  constraint vertical L1
  constraint midpoint L0 P2
  constraint coincident A2 P2
  constraint coincident P3 A3
  constraint coincident A4 P5
  constraint horizontal L2
  constraint coincident A4 P4
  constraint coincident P4 L3.end
  constraint coincident P5 L2.end
  constraint coincident P3 A5
  constraint coincident P4 A5
  constraint coincident L3 A5.centre
  constraint coincident L3 A7.centre
  constraint tangent A4 A7
  constraint tangent A6 A7
  constraint coincident P3 A8.end
  constraint coincident A5.centre A6.centre
  constraint coincident A3 A9.end
  constraint coincident A6 A9.end
  constraint coincident A6 P6
  constraint coincident A7 P6
  constraint coincident P6 A9.start
  constraint tangent A25 A26
  constraint tangent A6 A26
  constraint coincident A9.end A26
  constraint coincident A26 A32.end
  constraint coincident A25 A32.end
  constraint coincident A3 A32.start
  constraint tangent A68 A69
  constraint tangent A69 A70
  constraint tangent A70 A71
  constraint tangent A68 A71
  constraint coincident A2 A69.centre
  constraint symmetric L1 A71.centre A69.centre
  measures "d84_1" angle of L2 L3
  measures "d101_1" distance of A71.centre A69.centre
  measures "d102_1" distance of A68.start A69.end
extrude "Extrude5''" add sketch "Sketch3 (3)" against normal up to surface (0.8 mm away) contours A68 A69 A70 A71 | A78 A80 A81 A83 | A86 A88 A89 A91 | A94 A96 A97 A99 | A102 A104 A105 A107 | A110 A112 A113 A115 bodies 8 in component "LensCap_Pergear10mm"
extrude "Extrude6''" cut sketch "Sketch3 (3)" against normal up to surface (1 mm away) contours A68 A69 A70 A71 | A73 A74 A75 A76 | A77 A79 A82 A84 | A78 A80 A81 A83 | A85 A87 A90 A92 | A86 A88 A89 A91 | A93 A95 A98 A100 | A94 A96 A97 A99 | A101 A103 A106 A108 | A102 A104 A105 A107 | A109 A111 A114 A116 | A110 A112 A113 A115 bodies 9 in component "LensCap_Pergear10mm"
extrude "Extrude7'" add sketch "Sketch3 (3)" along normal up to surface (1 mm away) from surface at 0.2 contours A3 A7 A8 A9 | A7 | A3 A10 A11 A12 | A12 | A3 A63 A64 A65 | A65 | A3 A13 A14 A15 | A15 | A3 A58 A59 A60 | A60 | A3 A16 A17 A18 | A18 | A3 A53 A54 A55 | A55 | A3 A19 A20 A21 | A21 | A3 A48 A49 A50 | A50 | A3 A22 A23 A24 | A24 | A3 A43 A44 A45 | A45 | A3 A38 A39 A40 | A40 bodies 10 in component "LensCap_Pergear10mm"
extrude "Extrude8'" cut sketch "Sketch3 (3)" along normal up to surface (1 mm away) from surface at 0.2 contours A3 A27 A33 | A3 A26 | A3 A27 | A3 A26 A32 | A3 A28 A34 | A3 A67 | A3 A67 | A3 A28 | A3 A66 A67 | A3 A29 A35 | A3 A62 | A3 A29 | A3 A61 A62 | A3 A30 A36 | A3 A57 | A3 A30 | A3 A56 A57 | A3 A31 A37 | A3 A52 | A3 A31 | A3 A51 A52 | A3 A41 A42 | A3 A47 | A3 A42 | A3 A46 A47 picked at (20.2057, -1.8001) picked at (18.3987, 8.5439) picked at (11.6618, 16.5986) picked at (8.543, -18.3991) picked at (1.8001, 20.2057) picked at (-1.7935, -20.2064) picked at (-8.5439, 18.3987) picked at (-11.6631, -16.5977) picked at (-16.5991, 11.661) picked at (-18.397, -8.5476) picked at (-20.2062, 1.7944) bodies 10 in component "LensCap_Pergear10mm"
chamfer "Chamfer10''" distance 0.3 angle 45 1 edges at (-17.3413, -6.726, 2.7) on bodies 8 in component "LensCap_Pergear10mm"
chamfer "Chamfer7''" distance 0.15 angle 45 1 faces at (-3.2368, -17.4757, 0.2) on bodies 10 in component "LensCap_Pergear10mm"
chamfer "Chamfer8''" distance 0.25 angle 45 1 faces at (-17.8291, -18.0986, 0) on bodies 9 in component "LensCap_Pergear10mm"
chamfer "Chamfer11'" distance 0.25 angle 45 1 edges at (-17.3413, -6.726, -1) on bodies 9 in component "LensCap_Pergear10mm"
chamfer "Chamfer12'" distance 0.2 angle 45 1 edges at (-28.9021, -11.2101, -7) on bodies 9 in component "LensCap_Pergear10mm"
chamfer "Chamfer13'" distance 0.2 angle 45 1 edges at (-17.3413, -6.726, 1.2) on bodies 8 in component "LensCap_Pergear10mm"
chamfer "Chamfer15'" distance 0.4 angle 45 1 edges at (-22.7488, -8.8234, 0) on bodies 8 in component "LensCap_Pergear10mm"
move_body "Move1" [suppressed] in component "LensCap_Sony20mm_2"
move_body "Move2" [suppressed] in component "LensCap_Sony20mm_2"
move_body "Move1'" [suppressed] in component "Blob"
move_body "Move2'" [suppressed] in component "Blob"
chamfer "Chamfer16" [suppressed] in component "LensCap_Pergear10mm"
component "LensCap_Sony20mm" placed x (1, 0, 0) y (0, 1, 0) z (0, 0, 1) at (0, 0, 0)
component "Blob" placed x (1, 0, 0) y (0, 1, 0) z (0, 0, 1) at (0, 0, 1.2)
component "LensCap_Sony20mm_2" placed x (1, 0, 0) y (0, 1, 0) z (0, 0, 1) at (0, 0, 0)
component "LensCap_Pergear10mm" placed x (1, 0, 0) y (0, 1, 0) z (0, 0, 1) at (0, 0, 0)
equation "d17 = 1 mm + 0.2 mm + 1.5 mm"
equation "d21 = ( 33.10 / 2 ) * 1 mm"
equation "d36 = ( 47.30 / 2 ) * 1 mm"
equation "d40 = ( 52 / 2 ) * 1 mm"
equation "d686 = ( 33 / 2 ) * 1 mm"
equation "d17_1 = 1 mm + 0.2 mm + 1.5 mm"
equation "d21_1 = ( ( 33 - 0.4 ) / 2 ) * 1 mm"
equation "d40_1 = ( 58 / 2 ) * 1 mm"
equation "d77 = ( 53.30 / 2 ) * 1 mm"
equation "d17_1_1 = 1 mm + 0.2 mm + 1.5 mm"
equation "d21_1_1 = ( ( 33 - 0.4 ) / 2 ) * 1 mm"
equation "d77_1 = ( 58 / 2 ) * 1 mm"
named bodies: "LC_Outer", "LC_Inner", "LC_Ring"
